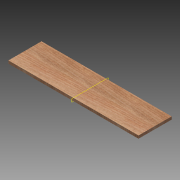
# Autodesk Inventor part: Generic Tail 1
Saved by Autodesk Inventor 2015 (Build 190159000, 159)
## iProperties
Created: 2018-07-21
Part Number: Generic Tail 1
Material: Wood (Birch)
Document SubType Name: Modeling
Designer: Michael Gunderman
Density: 0.401284 g/cm^3
Appearance: Birch - Natural Polished
Mass: 750 g
Surface Area: 2755.4 cm^2
Volume: 1869 cm^3
Author: Michael Gunderman
Autodesk Inventor part; units mm, degrees
ref_plane "XZ Plane" through (0, 0, 0) normal (0, 1, 0) x (-1, 0, 0)
ref_plane "XY Plane" through (0, 0, 0) normal (0, 0, 1) x (1, 0, 0)
sketch "Sketch1" plane through (0, 0, 0) normal (0, 1, 0) x (-1, 0, 0)
  line L0 (0, 0) -> (0, 178)
  line L1 (0, 178) -> (700, 178)
  line L2 (700, 178) -> (700, 0)
  line L3 (700, 0) -> (0, 0)
  dimension "d0" = 178
  dimension "d1" = 700
  constraints: 8 end point, 3 perpendicular, 1 vertical
  measures "d0" distance of L0.start L0.end
  measures "d1" distance of L0.end L1.end
extrude "Extrusion1" add sketch "Sketch1" along normal blind 15
ref_plane "Work Plane1" through (-350, 0, 0) normal (1, 0, 0) x (0, 1, 0)
body "Solid1"
